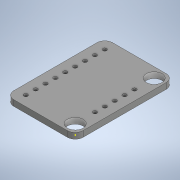
# Autodesk Inventor part: Adafruit_IMU
Saved by Autodesk Inventor 2020.3 (Build 243373000, 373)
## iProperties
Created: 2021-03-18
Part Number: Adafruit_IMU
Material: Ogólny
Document SubType Name: Modeling
Designer: patry
Density: 1 g/cm^3
Appearance: Domyślna
Author: patry
Autodesk Inventor part; units mm, degrees
ref_plane "YZ Plane" through (0, 0, 0) normal (1, 0, 0) x (0, 1, 0)
ref_plane "XZ Plane" through (0, 0, 0) normal (0, 1, 0) x (-1, 0, 0)
ref_plane "XY Plane" through (0, 0, 0) normal (0, 0, 1) x (1, 0, 0)
sketch "Szkic1" plane through (0, 0, 0) normal (0, 1, 0) x (-1, 0, 0)
  line L0 (2, 0) -> (15.8, 0)
  line L1 (17.8, -2) -> (17.8, -23.4)
  line L2 (15.8, -25.4) -> (2, -25.4)
  line L3 (0, -23.4) -> (0, -2)
  arc A0 (17.8, -2) -> (15.8, 0) centre (15.8, -2) ccw
  arc A1 (15.8, -25.4) -> (17.8, -23.4) centre (15.8, -23.4) ccw
  arc A2 (0, -23.4) -> (2, -25.4) centre (2, -23.4) ccw
  arc A3 (2, 0) -> (0, -2) centre (2, -2) ccw
  point P0 (0, 0)
  point P1 (17.8, -25.4)
  point P2 (17.8, 0)
  point P3 (0, -25.4)
  dimension "d0" = 17.8
  dimension "d1" = 25.4
  dimension "d2" = 2
  constraints: 8 end point, 8 point on circle, 8 point on line, 8 tangent, 4 centre point, 3 equal radius, 2 parallel, 1 horizontal, 1 perpendicular
  measures "d0" distance of point (17.8, -25.4) point (0, -25.4)
  measures "d1" distance of point (17.8, 0) point (17.8, -25.4)
  measures "d2" radius of A0
extrude "Wyciągnięcie proste1" add sketch "Szkic1" along normal blind 1.5
sketch "Szkic2" plane through (0, 1.5, 0) normal (0, 1, 0) x (1, 0, 0)
  line L0 (-2, 25.4) -> (-15.8, 25.4) projected
  line L1 (-17.8, 23.4) -> (-17.8, 2) projected
  line L2 (0, 2) -> (0, 23.4) projected
  point P0 (0, 0)
  point P1 (-2.54, 7.62)
  point P2 (-2.54, 10.16)
  point P3 (-2.54, 12.7)
  point P4 (-2.54, 15.24)
  point P5 (-2.54, 17.78)
  point P6 (-15.26, 2.54)
  point P7 (-15.26, 5.08)
  point P8 (-15.26, 7.62)
  point P9 (-15.26, 10.16)
  point P10 (-15.26, 12.7)
  point P11 (-15.26, 15.24)
  point P12 (-15.26, 17.78)
  point P13 (-15.26, 20.32)
  point P14 (-15.26, 22.86)
  dimension "d5" = 2.54
  dimension "d6" = 2.54
  dimension "d7" = 2.54
  dimension "d8" = 2.54
  dimension "d9" = 2.54
  dimension "d10" = 2.54
  dimension "d11" = 2.54
  dimension "d12" = 2.54
  dimension "d13" = 2.54
  dimension "d14" = 2.54
  dimension "d15" = 2.54
  dimension "d16" = 2.54
  dimension "d17" = 2.54
  dimension "d18" = 2.54
  dimension "d19" = 2.54
  constraints: 12 vertical alignment, 1 horizontal alignment
  measures "d5" distance of point (-15.26, 5.08) point (-15.26, 2.54)
  measures "d6" distance of point (-15.26, 7.62) point (-15.26, 5.08)
  measures "d7" distance of point (-15.26, 10.16) point (-15.26, 7.62)
  measures "d8" distance of point (-15.26, 12.7) point (-15.26, 10.16)
  measures "d9" distance of point (-15.26, 15.24) point (-15.26, 12.7)
  measures "d10" distance of point (-15.26, 17.78) point (-15.26, 15.24)
  measures "d11" distance of point (-15.26, 20.32) point (-15.26, 17.78)
  measures "d12" distance of point (-15.26, 22.86) point (-15.26, 20.32)
  measures "d13" distance from line of L0 point (-15.26, 22.86)
  measures "d14" distance from line of L1 point (-15.26, 12.7)
  measures "d15" distance of point (-2.54, 15.24) point (-2.54, 17.78)
  measures "d16" distance of point (-2.54, 12.7) point (-2.54, 15.24)
  measures "d17" distance of point (-2.54, 10.16) point (-2.54, 12.7)
  measures "d18" distance of point (-2.54, 7.62) point (-2.54, 10.16)
  measures "d19" distance from line of L2 point (-2.54, 17.78)
hole "Otwór1" at (-2.54, 1.5, -7.62) at (-2.54, 1.5, -10.16) at (-2.54, 1.5, -12.7) at (-2.54, 1.5, -15.24) at (-2.54, 1.5, -17.78) at (-15.26, 1.5, -2.54) at (-15.26, 1.5, -5.08) at (-15.26, 1.5, -7.62) at (-15.26, 1.5, -10.16) at (-15.26, 1.5, -12.7) at (-15.26, 1.5, -15.24) at (-15.26, 1.5, -17.78) at (-15.26, 1.5, -20.32) at (-15.26, 1.5, -22.86) direction (0, -1, 0) diameter 1 end through all
sketch "Szkic3" plane through (0, 1.5, 0) normal (0, 1, 0) x (1, 0, 0)
  point P0 (0, 0)
sketch "Szkic4" plane through (0, 1.5, 0) normal (0, 1, 0) x (1, 0, 0)
  circle A0 centre (-2.54, 17.78) radius 0.5 construction
  circle A1 centre (-2.54, 7.62) radius 0.5 construction
  line L0 (-2.54, 17.78) -> (-2.54, 7.62) construction
  line L1 (-2.54, 17.78) -> (-2.54, -1.5246) construction
  circle A2 centre (-2.54, 12.7) radius 0.5 construction
  line L2 (-2.54, 12.7) -> (-2.54, 26.7995) construction
  circle A3 centre (-2.54, 22.86) radius 2
  line L3 (-2, 25.4) -> (-15.8, 25.4) projected
  circle A4 centre (-2.54, 2.54) radius 2
  line L4 (-15.8, 0) -> (-2, 0) projected
  point P0 (0, 0)
  dimension "d27" = 4
  dimension "d28" = 2.54
  dimension "d29" = 4
  dimension "d30" = 2.54
  constraints: 6 end point, 3 vertical, 2 centre point, 2 point on line
  measures "d27" diameter of A3
  measures "d28" distance from line of L3 A3.centre
  measures "d29" diameter of A4
  measures "d30" distance from line of L4 A4.centre
extrude "Wyciągnięcie proste2" cut sketch "Szkic4" against normal blind 10
equation "\"d6\" = d5"
equation "\"d7\" = d6"
equation "\"d8\" = d7"
equation "\"d9\" = d8"
equation "\"d10\" = d9"
equation "\"d11\" = d10"
equation "\"d12\" = d11"
equation "\"d13\" = d12"
equation "\"d14\" = d8"
equation "\"d16\" = d15"
equation "\"d17\" = d16"
equation "\"d18\" = d17"
